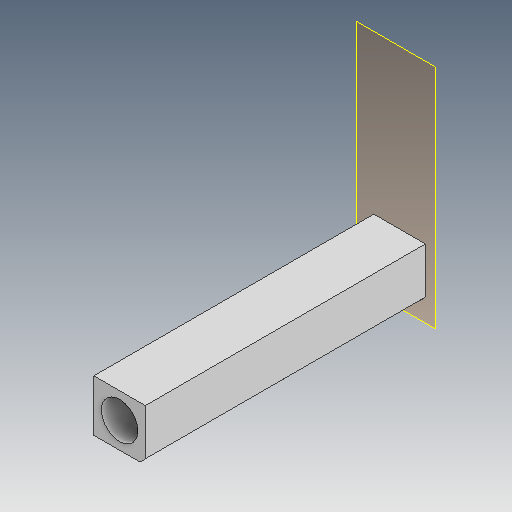
# Autodesk Inventor part: odometry standoff
Saved by Autodesk Inventor 2020 (Build 240168000, 168)
## iProperties
Created: 2019-11-23
Part Number: odometry standoff
Material: Generic
Document SubType Name: Modeling
Designer: ball
Density: 1 g/cm^3
Appearance: Default
Author: ball
Autodesk Inventor part; units mm, degrees
ref_plane "YZ Plane" through (0, 0, 0) normal (1, 0, 0) x (0, 1, 0)
ref_plane "XZ Plane" through (0, 0, 0) normal (0, 1, 0) x (-1, 0, 0)
ref_plane "Work Plane1" through (0, 0, 0) normal (0, 0, 1) x (1, 0, 0)
sketch "Sketch1" plane through (0, 0, 0) normal (0, 0, 1) x (1, 0, 0)
  circle A0 centre (0.445, -8.7) radius 2.25 construction
  circle A1 centre (0.445, -8.7) radius 2.25
  line L0 (3.62, -5.525) -> (-2.73, -5.525)
  line L1 (-2.73, -5.525) -> (-2.73, -11.875)
  line L2 (3.62, -5.525) -> (-2.73, -11.875) construction
  arc A2 (1.27, -12.7) -> (4.445, -9.525) centre (1.27, -9.525) ccw construction
  arc A3 (2.9413, -11.875) -> (3.62, -11.1963) centre (0.445, -8.7) ccw
  line L3 (3.62, -11.1963) -> (3.62, -5.525)
  line L4 (-2.73, -11.875) -> (2.9413, -11.875)
  point P0 (0, 0)
  dimension "d1" = 6.35
  constraints: 10 end point, 2 centre point, 2 coincident, 2 parallel, 2 point on circle, 1 concentric, 1 horizontal, 1 midpoint, 1 perpendicular
  measures "d1" distance of L1.end L0.end
ref_plane "Work Plane2" through (-350.7586, -218.6666, 34.497) normal (0, 0, -1) x (-0.0253, 0.9997, 0)
extrude "Extrusion1" add sketch "Sketch1" along normal up to surface (34.497 mm away)
body "Solid1"
